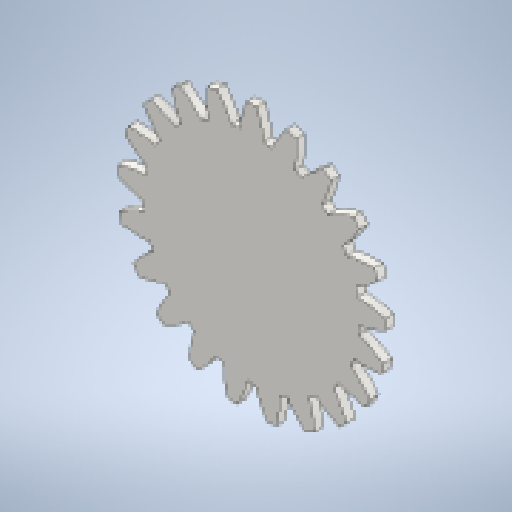
# Autodesk Inventor part: 平歯車1
Saved by Autodesk Inventor 2024 (Build 280153000, 153)
## iProperties
Created: 2024-06-08
Part Number: 平歯車1
Material: Steel
Document SubType Name: Modeling
Designer: right
Categories: <?xml version="1.0" encoding="UTF-16"?> <MemberInstance><Categories><FamilyTemplate><FamilyTemplateParameter ValueType="xs:double" Id="1" ObjectReferenceKey="da_z" ObjectType="kUserParameterObject"/><FamilyTemplateParameter ValueType="xs:double" Id="2" ObjectReferenceKey="da_b" ObjectType="kUserParameterObject"/><FamilyTemplateParameter ValueType="xs:double" Id="3" ObjectReferenceKey="da_beta" ObjectType="kUserParameterObject"/><FamilyTemplateParameter ValueType="xs:double" Id="4" ObjectReferenceKey="da_da" ObjectType="kUserParameterObject"/><FamilyTemplateParameter ValueType="xs:double" Id="5" ObjectReferenceKey="da_aw" ObjectType="kUserParameterObject"/><FamilyTemplateParameter ValueType="xs:string" Id="6" ObjectReferenceKey="EAIAABAAAACIAQAAAAAAAIAAAAAAAAAA" ObjectType="83910656" SubObjectId="SurfaceGeometry"/></FamilyTemplate><ParamToTemplateMap><ParamToTemplate CategoryParameter="//CategoryParameter[@InternalName='046C89C9-8512-4d59-83FE-43B91F4F132A']" TemplateParameter="1"/><ParamToTemplate CategoryParameter="//CategoryParameter[@InternalName='2552DF32-E462-4b46-AEBF-C6C7768E72AC']" TemplateParameter="2"/><ParamToTemplate CategoryParameter="//CategoryParameter[@InternalName='C9EE641D-15FC-4fae-A226-E94C4372FDD7']" TemplateParameter="3"/><ParamToTemplate><ParamToTemplate CategoryParameter="//CategoryParameter[@InternalName='00B6519A-459B-49c7-AD84-2E56D39A5744']" ConstantValue="0.035417"/></ParamToTemplate><ParamToTemplate><ParamToTemplate CategoryParameter="//CategoryParameter[@InternalName='04B31F0E-C7A6-4894-AA32-9629BEFACF47']" ConstantValue="1.000000"/></ParamToTemplate><ParamToTemplate><ParamToTemplate CategoryParameter="//CategoryParameter[@InternalName='43CBEC2E-7847-49e7-A936-2F7889FCB2D9']" ConstantValue="0.250000"/></ParamToTemplate><ParamToTemplate><ParamToTemplate CategoryParameter="//CategoryParameter[@InternalName='B1EFC894-105D-4ebd-86BF-FA20ED196853']" ConstantValue="0.350000"/></ParamToTemplate><ParamToTemplate><ParamToTemplate CategoryParameter="//CategoryParameter[@InternalName='51175063-3D10-4879-93E8-6246FE8B403D']" ConstantValue="2060000000.000000"/></ParamToTemplate><ParamToTemplate><ParamToTemplate CategoryParameter="//CategoryParameter[@InternalName='A3A52E27-4454-46a9-B0BD-C932399B70AF']" ConstantValue="0.300000"/></ParamToTemplate><ParamToTemplate><ParamToTemplate CategoryParameter="//CategoryParameter[@InternalName='91B76062-C214-41d9-B1B9-14D2AB99603D']" ConstantValue="0.400000"/></ParamToTemplate><ParamToTemplate><ParamToTemplate CategoryParameter="//CategoryParameter[@InternalName='374E806E-8B8A-4dda-A9AA-1039D6500AD2']" ConstantValue="2.500000"/></ParamToTemplate><ParamToTemplate><ParamToTemplate CategoryParameter="//CategoryParameter[@InternalName='2D373A89-B862-43d6-8D0B-0CBF12AB9F6C']" ConstantValue="0.349066"/></ParamToTemplate><ParamToTemplate CategoryParameter="//CategoryParameter[@InternalName='37777632-D6A2-4fac-9D53-DB8ACD95C989']" TemplateParameter="4"/><ParamToTemplate CategoryParameter="//CategoryParameter[@InternalName='FD1017F1-B727-4f7e-9707-0F86F1FF9423']" TemplateParameter="5"/><ParamToTemplate><ParamToTemplate CategoryParameter="//CategoryParameter[@InternalName='9E1B4470-B2D3-4ff1-B813-535BB4CDF51A']" ConstantValue="3520000.000000"/></ParamToTemplate><ParamToTemplate><ParamToTemplate CategoryParameter="//CategoryParameter[@InternalName='F8452263-BFF6-458c-9FB1-07C4B99E95CD']" ConstantValue="11400000.000000"/></ParamToTemplate><ParamToTemplate><ParamToTemplate CategoryParameter="//CategoryParameter[@InternalName='3E3BB259-FD49-497f-8171-6EBC954A3479']" ConstantValue="2.000000"/></ParamToTemplate><ParamToTemplate CategoryParameter="//CategoryParameter[@InternalName='27C3BAF2-7550-4e4b-AE2C-0DB134B7D9B7']" TemplateParameter="6"/></ParamToTemplateMap><Category DisplayName="Gear" InternalName="DC85795E-93AB-48d5-8EEE-5A27447B64BD" Mnemonic="Gear"><CategoryParameter DisplayName="z" InternalName="046C89C9-8512-4d59-83FE-43B91F4F132A" Mnemonic="z"/><CategoryParameter DisplayName="b" InternalName="2552DF32-E462-4b46-AEBF-C6C7768E72AC" Mnemonic="b"/><CategoryParameter DisplayName="||b|" InternalName="C9EE641D-15FC-4fae-A226-E94C4372FDD7" Mnemonic="beta"/><CategoryParameter DisplayName="x" InternalName="00B6519A-459B-49c7-AD84-2E56D39A5744" Mnemonic="x"/><CategoryParameter DisplayName="a*" InternalName="04B31F0E-C7A6-4894-AA32-9629BEFACF47" Mnemonic="a"/><CategoryParameter DisplayName="c*" InternalName="43CBEC2E-7847-49e7-A936-2F7889FCB2D9" Mnemonic="c"/><CategoryParameter DisplayName="r|.f|*" InternalName="B1EFC894-105D-4ebd-86BF-FA20ED196853" Mnemonic="rf"/><CategoryParameter DisplayName="E" InternalName="51175063-3D10-4879-93E8-6246FE8B403D" Mnemonic="E"/><CategoryParameter DisplayName="||m|" InternalName="A3A52E27-4454-46a9-B0BD-C932399B70AF" Mnemonic="mi"/><Category DisplayName="SpurGear" InternalName="26C5A22E-A91E-4dfd-A3B3-23CCAFAE1764" Mnemonic="SpurGear"><CategoryParameter DisplayName="m" InternalName="91B76062-C214-41d9-B1B9-14D2AB99603D" Mnemonic="m"/><CategoryParameter DisplayName="P" InternalName="374E806E-8B8A-4dda-A9AA-1039D6500AD2" Mnemonic="PP"/><CategoryParameter DisplayName="||a|" InternalName="2D373A89-B862-43d6-8D0B-0CBF12AB9F6C" Mnemonic="alpha"/><CategoryParameter DisplayName="d|.a|" InternalName="37777632-D6A2-4fac-9D53-DB8ACD95C989" Mnemonic="da"/><CategoryParameter DisplayName="a|.w|" InternalName="FD1017F1-B727-4f7e-9707-0F86F1FF9423" Mnemonic="aw"/><CategoryParameter DisplayName="||s||.Flim|" InternalName="9E1B4470-B2D3-4ff1-B813-535BB4CDF51A" Mnemonic="sFlim"/><CategoryParameter DisplayName="||s||.Hlim|" InternalName="F8452263-BFF6-458c-9FB1-07C4B99E95CD" Mnemonic="sHlim"/><CategoryParameter DisplayName="タイプ" InternalName="3E3BB259-FD49-497f-8171-6EBC954A3479" Mnemonic="type"/><CategoryParameter DisplayName="PitchDiameter" InternalName="27C3BAF2-7550-4e4b-AE2C-0DB134B7D9B7" Mnemonic="IDS_PITCHDIAM"/></Category></Category></Categories></MemberInstance>
Density: 1 g/cm^3
Appearance: Steel
CustomPartVersion: 1
Author: right
Autodesk Inventor part; units mm, degrees
sketch "Sketch1" plane through (0, 0, 0) normal (0, 0, 1) x (1, 0, 0)
  circle A0 centre (0, 0) radius 46.1417
  dimension "d0" = 92.2833
  constraints: 1 centre point
  measures "d0" diameter of A0
extrude "Extrusion1" add sketch "Sketch1" along normal blind 30
ref_plane "Work Plane2" through (0, 0, 15) normal (0, 0, 1) x (1, 0, 0)
sketch "Sketch2" plane through (0, 0, 0) normal (0, 0, -1) x (-1, 0, 0)
  circle A0 centre (0, 0) radius 46.1417 projected
  circle A1 centre (0, 0) radius 42
  dimension "d3" = 84
  constraints: 1 centre point, 1 coincident
  measures "d3" diameter of A1
surface extrude "ピッチ円直径" sketch "Sketch2" against normal through all shown no curves A1
ref_plane "Work Plane8" through (0, 0, 0) normal (0.9888308, 0.1490423, 0) x (0, 0, 1)
ref_plane "Work Plane9" through (0, 0, 0) normal (1, 0, 0) x (0, 1, 0)
spur gear teeth "平歯車" teeth 21 pitch diameter 84 tip diameter 92.2833 root diameter 74.2833 face width 30 start plane through (0, 0, 0) normal (0, 0, -1) x (-1, 0, 0)
sketch "スケッチ3" plane through (0, 0, 30) normal (0, 0, 1) x (1, 0, 0)
  arc A0 (-15.2396, 43.5524) -> (-14.8527, 34.0427) centre (18.5549, 40.1648) ccw projected
  arc A1 (-14.8527, 34.0427) -> (-17.3551, 32.8375) centre (0, 0) ccw projected
  arc A2 (-17.3551, 32.8375) -> (-24.5488, 39.0693) centre (-42.9709, 10.5356) ccw projected
  arc A3 (-24.5488, 39.0693) -> (-27.3999, 37.1255) centre (0, 0) ccw projected
  arc A4 (-27.3999, 37.1255) -> (-24.227, 28.1523) centre (5.8917, 43.8495) ccw projected
  arc A5 (-24.227, 28.1523) -> (-26.2631, 26.2631) centre (0, 0) ccw projected
  arc A6 (-26.2631, 26.2631) -> (-34.9741, 30.0976) centre (-44.1672, -2.5984) ccw projected
  arc A7 (-34.9741, 30.0976) -> (-37.1255, 27.3999) centre (0, 0) ccw projected
  arc A8 (-37.1255, 27.3999) -> (-31.4487, 19.7606) centre (-7.2949, 43.638) ccw projected
  arc A9 (-31.4487, 19.7606) -> (-32.8375, 17.3551) centre (0, 0) ccw projected
  arc A10 (-32.8375, 17.3551) -> (-42.2917, 18.4517) centre (-41.4391, -15.5015) ccw projected
  arc A11 (-42.2917, 18.4517) -> (-43.5524, 15.2396) centre (0, 0) ccw projected
  arc A12 (-43.5524, 15.2396) -> (-35.8761, 9.613) centre (-19.8333, 39.5491) ccw projected
  arc A13 (-35.8761, 9.613) -> (-36.4942, 6.9051) centre (0, 0) ccw projected
  arc A14 (-36.4942, 6.9051) -> (-45.8515, 5.1662) centre (-35.0289, -27.0272) ccw projected
  arc A15 (-45.8515, 5.1662) -> (-46.1094, 1.7253) centre (0, 0) ccw projected
  arc A16 (-46.1094, 1.7253) -> (-37.1157, -1.3888) centre (-30.6095, 31.9461) ccw projected
  arc A17 (-37.1157, -1.3888) -> (-36.9081, -4.1585) centre (0, 0) ccw projected
  arc A18 (-36.9081, -4.1585) -> (-45.3373, -8.5783) centre (-25.5063, -36.1514) ccw projected
  arc A19 (-45.3373, -8.5783) -> (-44.5694, -11.9423) centre (0, 0) ccw projected
  arc A20 (-44.5694, -11.9423) -> (-35.0574, -12.2671) centre (-38.6659, 21.5045) ccw projected
  arc A21 (-35.0574, -12.2671) -> (-34.0427, -14.8527) centre (0, 0) ccw projected
  arc A22 (-34.0427, -14.8527) -> (-40.7946, -21.5606) centre (-13.7173, -42.0634) ccw projected
  arc A23 (-40.7946, -21.5606) -> (-39.0693, -24.5488) centre (0, 0) ccw projected
  arc A24 (-39.0693, -24.5488) -> (-29.8841, -22.0555) centre (-43.2866, 9.1521) ccw projected
  arc A25 (-29.8841, -22.0555) -> (-28.1523, -24.227) centre (0, 0) ccw projected
  arc A26 (-28.1523, -24.227) -> (-32.6271, -32.6271) centre (-0.7095, -44.2379) ccw projected
  arc A27 (-32.6271, -32.6271) -> (-30.0976, -34.9741) centre (0, 0) ccw projected
  arc A28 (-30.0976, -34.9741) -> (-22.0555, -29.8841) centre (-44.0612, -4.0134) ccw projected
  arc A29 (-22.0555, -29.8841) -> (-19.7606, -31.4487) centre (0, 0) ccw projected
  arc A30 (-19.7606, -31.4487) -> (-21.5606, -40.7946) centre (12.3614, -42.4816) ccw projected
  arc A31 (-21.5606, -40.7946) -> (-18.4517, -42.2917) centre (0, 0) ccw projected
  arc A32 (-18.4517, -42.2917) -> (-12.2671, -35.0574) centre (-40.9207, -16.8224) ccw projected
  arc A33 (-12.2671, -35.0574) -> (-9.613, -35.8761) centre (0, 0) ccw projected
  arc A34 (-9.613, -35.8761) -> (-8.5783, -45.3373) centre (24.3339, -36.9507) ccw projected
  arc A35 (-8.5783, -45.3373) -> (-5.1662, -45.8515) centre (0, 0) ccw projected
  arc A36 (-5.1662, -45.8515) -> (-1.3888, -37.1157) centre (-34.1442, -28.1366) ccw projected
  arc A37 (-1.3888, -37.1157) -> (1.3888, -37.1157) centre (0, 0) ccw projected
  arc A38 (1.3888, -37.1157) -> (5.1662, -45.8515) centre (34.1442, -28.1366) ccw projected
  arc A39 (5.1662, -45.8515) -> (8.5783, -45.3373) centre (0, 0) ccw projected
  arc A40 (8.5783, -45.3373) -> (9.613, -35.8761) centre (-24.3339, -36.9507) ccw projected
  arc A41 (9.613, -35.8761) -> (12.2671, -35.0574) centre (0, 0) ccw projected
  arc A42 (12.2671, -35.0574) -> (18.4517, -42.2917) centre (40.9207, -16.8224) ccw projected
  arc A43 (18.4517, -42.2917) -> (21.5606, -40.7946) centre (0, 0) ccw projected
  arc A44 (21.5606, -40.7946) -> (19.7606, -31.4487) centre (-12.3614, -42.4816) ccw projected
  arc A45 (19.7606, -31.4487) -> (22.0555, -29.8841) centre (0, 0) ccw projected
  arc A46 (22.0555, -29.8841) -> (30.0976, -34.9741) centre (44.0612, -4.0134) ccw projected
  arc A47 (30.0976, -34.9741) -> (32.6271, -32.6271) centre (0, 0) ccw projected
  arc A48 (32.6271, -32.6271) -> (28.1523, -24.227) centre (0.7095, -44.2379) ccw projected
  arc A49 (28.1523, -24.227) -> (29.8841, -22.0555) centre (0, 0) ccw projected
  arc A50 (29.8841, -22.0555) -> (39.0693, -24.5488) centre (43.2866, 9.1521) ccw projected
  arc A51 (39.0693, -24.5488) -> (40.7946, -21.5606) centre (0, 0) ccw projected
  arc A52 (40.7946, -21.5606) -> (34.0427, -14.8527) centre (13.7173, -42.0634) ccw projected
  arc A53 (34.0427, -14.8527) -> (35.0574, -12.2671) centre (0, 0) ccw projected
  arc A54 (35.0574, -12.2671) -> (44.5694, -11.9423) centre (38.6659, 21.5045) ccw projected
  arc A55 (44.5694, -11.9423) -> (45.3373, -8.5783) centre (0, 0) ccw projected
  arc A56 (45.3373, -8.5783) -> (36.9081, -4.1585) centre (25.5063, -36.1514) ccw projected
  arc A57 (36.9081, -4.1585) -> (37.1157, -1.3888) centre (0, 0) ccw projected
  arc A58 (37.1157, -1.3888) -> (46.1094, 1.7253) centre (30.6095, 31.9461) ccw projected
  arc A59 (46.1094, 1.7253) -> (45.8515, 5.1662) centre (0, 0) ccw projected
  arc A60 (45.8515, 5.1662) -> (36.4942, 6.9051) centre (35.0289, -27.0272) ccw projected
  arc A61 (36.4942, 6.9051) -> (35.8761, 9.613) centre (0, 0) ccw projected
  arc A62 (35.8761, 9.613) -> (43.5524, 15.2396) centre (19.8333, 39.5491) ccw projected
  arc A63 (43.5524, 15.2396) -> (42.2917, 18.4517) centre (0, 0) ccw projected
  arc A64 (42.2917, 18.4517) -> (32.8375, 17.3551) centre (41.4391, -15.5015) ccw projected
  arc A65 (32.8375, 17.3551) -> (31.4487, 19.7606) centre (0, 0) ccw projected
  arc A66 (31.4487, 19.7606) -> (37.1255, 27.3999) centre (7.2949, 43.638) ccw projected
  arc A67 (37.1255, 27.3999) -> (34.9741, 30.0976) centre (0, 0) ccw projected
  arc A68 (34.9741, 30.0976) -> (26.2631, 26.2631) centre (44.1672, -2.5984) ccw projected
  arc A69 (26.2631, 26.2631) -> (24.227, 28.1523) centre (0, 0) ccw projected
  arc A70 (24.227, 28.1523) -> (27.3999, 37.1255) centre (-5.8917, 43.8495) ccw projected
  arc A71 (27.3999, 37.1255) -> (24.5488, 39.0693) centre (0, 0) ccw projected
  arc A72 (24.5488, 39.0693) -> (17.3551, 32.8375) centre (42.9709, 10.5356) ccw projected
  arc A73 (17.3551, 32.8375) -> (14.8527, 34.0427) centre (0, 0) ccw projected
  arc A74 (14.8527, 34.0427) -> (15.2396, 43.5524) centre (-18.5549, 40.1648) ccw projected
  arc A75 (15.2396, 43.5524) -> (11.9423, 44.5694) centre (0, 0) ccw projected
  arc A76 (11.9423, 44.5694) -> (6.9051, 36.4942) centre (37.9564, 22.7334) ccw projected
  arc A77 (6.9051, 36.4942) -> (4.1585, 36.9081) centre (0, 0) ccw projected
  arc A78 (4.1585, 36.9081) -> (1.7253, 46.1094) centre (-29.5693, 32.9112) ccw projected
  arc A79 (1.7253, 46.1094) -> (-1.7253, 46.1094) centre (0, 0) ccw projected
  arc A80 (-1.7253, 46.1094) -> (-4.1585, 36.9081) centre (29.5693, 32.9112) ccw projected
  arc A81 (-4.1585, 36.9081) -> (-6.9051, 36.4942) centre (0, 0) ccw projected
  arc A82 (-6.9051, 36.4942) -> (-11.9423, 44.5694) centre (-37.9564, 22.7334) ccw projected
  arc A83 (-11.9423, 44.5694) -> (-15.2396, 43.5524) centre (0, 0) ccw projected
extrude "押し出し2" cut sketch "スケッチ3" against normal blind 27
sketch "スケッチ4" plane through (0, 0, 3) normal (0, 0, 1) x (1, 0, 0)
  circle A0 centre (0, 0) radius 10
  circle A1 centre (0, 0) radius 7 construction
  circle A2 centre (0, 0) radius 5
  circle A3 centre (-7, 0) radius 1.1
  circle A4 centre (-4.9497, -4.9497) radius 1.1
  circle A5 centre (0, -7) radius 1.1
  circle A6 centre (4.9497, -4.9497) radius 1.1
  circle A7 centre (7, 0) radius 1.1
  circle A8 centre (4.9497, 4.9497) radius 1.1
  circle A9 centre (0, 7) radius 1.1
  circle A10 centre (-4.9497, 4.9497) radius 1.1
  arc A11 (-14.8527, 34.0427) -> (-17.3551, 32.8375) centre (0, 0) ccw projected
  arc A12 (-17.3551, 32.8375) -> (-24.5488, 39.0693) centre (-42.9709, 10.5356) ccw projected
  arc A13 (-24.5488, 39.0693) -> (-27.3999, 37.1255) centre (0, 0) ccw projected
  arc A14 (-27.3999, 37.1255) -> (-24.227, 28.1523) centre (5.8917, 43.8495) ccw projected
  arc A15 (-24.227, 28.1523) -> (-26.2631, 26.2631) centre (0, 0) ccw projected
  arc A16 (-26.2631, 26.2631) -> (-34.9741, 30.0976) centre (-44.1672, -2.5984) ccw projected
  arc A17 (-34.9741, 30.0976) -> (-37.1255, 27.3999) centre (0, 0) ccw projected
  arc A18 (-37.1255, 27.3999) -> (-31.4487, 19.7606) centre (-7.2949, 43.638) ccw projected
  arc A19 (-31.4487, 19.7606) -> (-32.8375, 17.3551) centre (0, 0) ccw projected
  arc A20 (-32.8375, 17.3551) -> (-42.2917, 18.4517) centre (-41.4391, -15.5015) ccw projected
  arc A21 (-42.2917, 18.4517) -> (-43.5524, 15.2396) centre (0, 0) ccw projected
  arc A22 (-43.5524, 15.2396) -> (-35.8761, 9.613) centre (-19.8333, 39.5491) ccw projected
  arc A23 (-35.8761, 9.613) -> (-36.4942, 6.9051) centre (0, 0) ccw projected
  arc A24 (-36.4942, 6.9051) -> (-45.8515, 5.1662) centre (-35.0289, -27.0272) ccw projected
  arc A25 (-45.8515, 5.1662) -> (-46.1094, 1.7253) centre (0, 0) ccw projected
  arc A26 (-46.1094, 1.7253) -> (-37.1157, -1.3888) centre (-30.6095, 31.9461) ccw projected
  arc A27 (-37.1157, -1.3888) -> (-36.9081, -4.1585) centre (0, 0) ccw projected
  arc A28 (-36.9081, -4.1585) -> (-45.3373, -8.5783) centre (-25.5063, -36.1514) ccw projected
  arc A29 (-45.3373, -8.5783) -> (-44.5694, -11.9423) centre (0, 0) ccw projected
  arc A30 (-44.5694, -11.9423) -> (-35.0574, -12.2671) centre (-38.6659, 21.5045) ccw projected
  arc A31 (-35.0574, -12.2671) -> (-34.0427, -14.8527) centre (0, 0) ccw projected
  arc A32 (-34.0427, -14.8527) -> (-40.7946, -21.5606) centre (-13.7173, -42.0634) ccw projected
  arc A33 (-40.7946, -21.5606) -> (-39.0693, -24.5488) centre (0, 0) ccw projected
  arc A34 (-39.0693, -24.5488) -> (-29.8841, -22.0555) centre (-43.2866, 9.1521) ccw projected
  arc A35 (-29.8841, -22.0555) -> (-28.1523, -24.227) centre (0, 0) ccw projected
  arc A36 (-28.1523, -24.227) -> (-32.6271, -32.6271) centre (-0.7095, -44.2379) ccw projected
  arc A37 (-32.6271, -32.6271) -> (-30.0976, -34.9741) centre (0, 0) ccw projected
  arc A38 (-30.0976, -34.9741) -> (-22.0555, -29.8841) centre (-44.0612, -4.0134) ccw projected
  arc A39 (-22.0555, -29.8841) -> (-19.7606, -31.4487) centre (0, 0) ccw projected
  arc A40 (-19.7606, -31.4487) -> (-21.5606, -40.7946) centre (12.3614, -42.4816) ccw projected
  arc A41 (-21.5606, -40.7946) -> (-18.4517, -42.2917) centre (0, 0) ccw projected
  arc A42 (-18.4517, -42.2917) -> (-12.2671, -35.0574) centre (-40.9207, -16.8224) ccw projected
  arc A43 (-12.2671, -35.0574) -> (-9.613, -35.8761) centre (0, 0) ccw projected
  arc A44 (-9.613, -35.8761) -> (-8.5783, -45.3373) centre (24.3339, -36.9507) ccw projected
  arc A45 (-8.5783, -45.3373) -> (-5.1662, -45.8515) centre (0, 0) ccw projected
  arc A46 (-5.1662, -45.8515) -> (-1.3888, -37.1157) centre (-34.1442, -28.1366) ccw projected
  arc A47 (-1.3888, -37.1157) -> (1.3888, -37.1157) centre (0, 0) ccw projected
  arc A48 (1.3888, -37.1157) -> (5.1662, -45.8515) centre (34.1442, -28.1366) ccw projected
  arc A49 (5.1662, -45.8515) -> (8.5783, -45.3373) centre (0, 0) ccw projected
  arc A50 (8.5783, -45.3373) -> (9.613, -35.8761) centre (-24.3339, -36.9507) ccw projected
  arc A51 (9.613, -35.8761) -> (12.2671, -35.0574) centre (0, 0) ccw projected
  arc A52 (12.2671, -35.0574) -> (18.4517, -42.2917) centre (40.9207, -16.8224) ccw projected
  arc A53 (18.4517, -42.2917) -> (21.5606, -40.7946) centre (0, 0) ccw projected
  arc A54 (21.5606, -40.7946) -> (19.7606, -31.4487) centre (-12.3614, -42.4816) ccw projected
  arc A55 (19.7606, -31.4487) -> (22.0555, -29.8841) centre (0, 0) ccw projected
  arc A56 (22.0555, -29.8841) -> (30.0976, -34.9741) centre (44.0612, -4.0134) ccw projected
  arc A57 (30.0976, -34.9741) -> (32.6271, -32.6271) centre (0, 0) ccw projected
  arc A58 (32.6271, -32.6271) -> (28.1523, -24.227) centre (0.7095, -44.2379) ccw projected
  arc A59 (28.1523, -24.227) -> (29.8841, -22.0555) centre (0, 0) ccw projected
  arc A60 (29.8841, -22.0555) -> (39.0693, -24.5488) centre (43.2866, 9.1521) ccw projected
  arc A61 (39.0693, -24.5488) -> (40.7946, -21.5606) centre (0, 0) ccw projected
  arc A62 (40.7946, -21.5606) -> (34.0427, -14.8527) centre (13.7173, -42.0634) ccw projected
  arc A63 (34.0427, -14.8527) -> (35.0574, -12.2671) centre (0, 0) ccw projected
  arc A64 (35.0574, -12.2671) -> (44.5694, -11.9423) centre (38.6659, 21.5045) ccw projected
  arc A65 (44.5694, -11.9423) -> (45.3373, -8.5783) centre (0, 0) ccw projected
  arc A66 (45.3373, -8.5783) -> (36.9081, -4.1585) centre (25.5063, -36.1514) ccw projected
  arc A67 (36.9081, -4.1585) -> (37.1157, -1.3888) centre (0, 0) ccw projected
  arc A68 (37.1157, -1.3888) -> (46.1094, 1.7253) centre (30.6095, 31.9461) ccw projected
  arc A69 (46.1094, 1.7253) -> (45.8515, 5.1662) centre (0, 0) ccw projected
  arc A70 (45.8515, 5.1662) -> (36.4942, 6.9051) centre (35.0289, -27.0272) ccw projected
  arc A71 (36.4942, 6.9051) -> (35.8761, 9.613) centre (0, 0) ccw projected
  arc A72 (35.8761, 9.613) -> (43.5524, 15.2396) centre (19.8333, 39.5491) ccw projected
  arc A73 (43.5524, 15.2396) -> (42.2917, 18.4517) centre (0, 0) ccw projected
  arc A74 (42.2917, 18.4517) -> (32.8375, 17.3551) centre (41.4391, -15.5015) ccw projected
  arc A75 (32.8375, 17.3551) -> (31.4487, 19.7606) centre (0, 0) ccw projected
  arc A76 (31.4487, 19.7606) -> (37.1255, 27.3999) centre (7.2949, 43.638) ccw projected
  arc A77 (37.1255, 27.3999) -> (34.9741, 30.0976) centre (0, 0) ccw projected
  arc A78 (34.9741, 30.0976) -> (26.2631, 26.2631) centre (44.1672, -2.5984) ccw projected
  arc A79 (26.2631, 26.2631) -> (24.227, 28.1523) centre (0, 0) ccw projected
  arc A80 (24.227, 28.1523) -> (27.3999, 37.1255) centre (-5.8917, 43.8495) ccw projected
  arc A81 (27.3999, 37.1255) -> (24.5488, 39.0693) centre (0, 0) ccw projected
  arc A82 (24.5488, 39.0693) -> (17.3551, 32.8375) centre (42.9709, 10.5356) ccw projected
  arc A83 (17.3551, 32.8375) -> (14.8527, 34.0427) centre (0, 0) ccw projected
  arc A84 (14.8527, 34.0427) -> (15.2396, 43.5524) centre (-18.5549, 40.1648) ccw projected
  arc A85 (15.2396, 43.5524) -> (11.9423, 44.5694) centre (0, 0) ccw projected
  arc A86 (11.9423, 44.5694) -> (6.9051, 36.4942) centre (37.9564, 22.7334) ccw projected
  arc A87 (6.9051, 36.4942) -> (4.1585, 36.9081) centre (0, 0) ccw projected
  arc A88 (4.1585, 36.9081) -> (1.7253, 46.1094) centre (-29.5693, 32.9112) ccw projected
  arc A89 (1.7253, 46.1094) -> (-1.7253, 46.1094) centre (0, 0) ccw projected
  arc A90 (-1.7253, 46.1094) -> (-4.1585, 36.9081) centre (29.5693, 32.9112) ccw projected
  arc A91 (-4.1585, 36.9081) -> (-6.9051, 36.4942) centre (0, 0) ccw projected
  arc A92 (-6.9051, 36.4942) -> (-11.9423, 44.5694) centre (-37.9564, 22.7334) ccw projected
  arc A93 (-11.9423, 44.5694) -> (-15.2396, 43.5524) centre (0, 0) ccw projected
  arc A94 (-15.2396, 43.5524) -> (-14.8527, 34.0427) centre (18.5549, 40.1648) ccw projected
  circle A95 centre (0, 0) radius 37.1417
  line L0 (37.1114, -1.5) -> (-37.1114, -1.5)
  line L1 (-37.1114, -1.5) -> (-37.1114, 1.5)
  line L2 (-37.1114, 1.5) -> (37.1114, 1.5)
  line L3 (37.1114, 1.5) -> (37.1114, -1.5)
  line L4 (37.1114, -1.5) -> (-37.1114, 1.5) construction
  line L5 (-37.1114, -1.5) -> (37.1114, 1.5) construction
  line L6 (-19.8547, -31.3894) -> (17.2566, 32.8894)
  line L7 (19.8547, 31.3894) -> (-17.2566, -32.8894)
  line L8 (17.2566, -32.8894) -> (-19.8547, 31.3894)
  line L9 (-17.2566, 32.8894) -> (19.8547, -31.3894)
  line L10 (37.1114, -1.5) -> (-37.1114, -1.5)
  line L11 (-37.1114, 1.5) -> (37.1114, 1.5)
  line L12 (19.8547, 31.3894) -> (-17.2566, -32.8894)
  line L13 (-19.8547, -31.3894) -> (17.2566, 32.8894)
  line L14 (-17.2566, 32.8894) -> (19.8547, -31.3894)
  line L15 (17.2566, -32.8894) -> (-19.8547, 31.3894)
  circle A96 centre (0, 0) radius 34.1417
  point P0 (-34.1087, -1.5)
  point P1 (-18.3534, -28.789)
  point P2 (-6.2425, -7.8123)
  point P3 (-9.8869, -1.5)
  point P4 (-18.3534, 28.789)
  point P5 (-34.1087, 1.5)
  point P6 (-9.8869, 1.5)
  point P7 (-6.2425, 7.8123)
  point P8 (15.7553, 30.289)
  point P9 (-15.7553, 30.289)
  point P10 (-3.6444, 9.3123)
  point P11 (3.6444, 9.3123)
  point P12 (34.1087, 1.5)
  point P13 (18.3534, 28.789)
  point P14 (6.2425, 7.8123)
  point P15 (9.8869, 1.5)
  point P16 (18.3534, -28.789)
  point P17 (34.1087, -1.5)
  point P18 (9.8869, -1.5)
  point P19 (6.2425, -7.8123)
  point P20 (-15.7553, -30.289)
  point P21 (15.7553, -30.289)
  point P22 (3.6444, -9.3123)
  point P23 (-3.6444, -9.3123)
  dimension "d52" = 14
  dimension "d51" = 20
  dimension "d53" = 10
  dimension "d54" = 2.2
  dimension "d57" = 360
  dimension "d59" = 3
  dimension "d62" = 360
  dimension "d64" = 3
  constraints: 32 end point, 12 centre point, 4 coincident, 2 horizontal alignment, 2 midpoint, 2 parallel, 2 point on circle, 1 horizontal, 1 perpendicular, 56 other
  measures "d51" diameter of A0
  measures "d53" diameter of A2
  measures "d54" diameter of A3
  measures "d59" distance between parallel lines of L0 L2
  measures "d64" radial gap between concentric circles of A95 A96
extrude "押し出し3" cut sketch "スケッチ4" against normal through all contours A0 L7 A96 L2 | L0 A96 L9 A0 | L2 L7 A2 | A2 L0 L9 L7 L2 | A2 L9 L0 | A0 L9 A96 L6 | L7 A8 | A8 L7 | L7 L2 L9 L6 A2 | L7 L9 L2 | L8 A96 L7 A0 | L9 A6 | A6 L9 | A2 L8 L7 L0 L9 | L0 L7 L9 | L6 L9 A2 | L9 L7 L0 L8 L6 L2 | L2 L6 L9 | A2 L7 L8 | L7 L8 L0 | A0 L2 A96 L8 | L9 L6 L2 L8 A2 | L6 L8 L2 | L6 A96 L0 A0 | A2 L6 L0 L8 L7 | L0 L6 L8 | L8 A10 | A10 L8 | L8 L2 A2 | L8 L6 L0 A2 L2 | L6 A4 | A4 L6 | A2 L0 L6 | A3 | A5 | A7 | A9
fillet "フィレット1" radius 2 24 edges at (-15.7553, -30.289, 1.5) (-18.3534, -28.789, 1.5) (-34.1087, -1.5, 1.5) (-34.1087, 1.5, 1.5) (-18.3534, 28.789, 1.5) (-15.7553, 30.289, 1.5) (15.7553, 30.289, 1.5) (18.3534, 28.789, 1.5) (34.1087, 1.5, 1.5) (34.1087, -1.5, 1.5) (18.3534, -28.789, 1.5) (15.7553, -30.289, 1.5) (-3.6444, -9.3123, 1.5) (-6.2425, -7.8123, 1.5) (6.2425, -7.8123, 1.5) (3.6444, -9.3123, 1.5) (-9.8869, -1.5, 1.5) (-9.8869, 1.5, 1.5) (-6.2425, 7.8123, 1.5) (-3.6444, 9.3123, 1.5) (3.6444, 9.3123, 1.5) (6.2425, 7.8123, 1.5) (9.8869, 1.5, 1.5) (9.8869, -1.5, 1.5)
sketch "スケッチ6" plane through (0, 0, 3) normal (0, 0, 1) x (1, 0, 0)
  circle A0 centre (0, 0) radius 41.7224
  arc A1 (45.8515, 5.1662) -> (36.4942, 6.9051) centre (35.0289, -27.0272) ccw projected
  arc A2 (36.9081, -4.1585) -> (37.1157, -1.3888) centre (0, 0) ccw projected
  line L0 (36.4942, 6.9051) -> (37.1157, -1.3888)
  arc A3 (46.1094, 1.7253) -> (45.8515, 5.1662) centre (0, 0) ccw projected
  line L1 (45.8515, 5.1662) -> (46.1094, 1.7253)
  point P0 (41.6058, 3.1179)
  point P1 (41.2341, 6.365)
  constraints: 4 end point, 3 point on circle, 1 centre point, 1 coincident
equation "\"d0\" = da_da"
equation "\"d1\" = da_b"
equation "\"d3\" = da_d"
equation "\"d16\" = da_aw"
equation "\"d43\" = da_aw"
equation "\"d46\" = da_aw"
equation "\"da_da\" = 92.283334"
equation "\"da_b\" = 30"
equation "\"da_d\" = 84"
equation "\"da_aw\" = 86"
body "Solid1"
body "Srf1"
